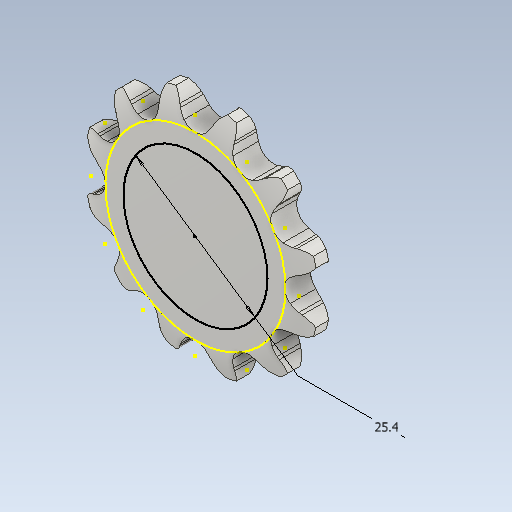
# Autodesk Inventor part: Roller Chain Sprocket2
Saved by Autodesk Inventor 2020 (Build 240168000, 168)
## iProperties
CustomPartVersion: 1
Created: 2021-01-13
Part Number: Roller Chain Sprocket2
Material: Steel
Document SubType Name: Modeling
Designer: lucky
Density: 7.85 g/cm^3
Appearance: Steel
Mass: 35.6372 g
Surface Area: 27.1032 cm^2
Volume: 4.53977 cm^3
Author: lucky
Autodesk Inventor part; units mm, degrees
ref_plane "YZ Plane" through (0, 0, 0) normal (1, 0, 0) x (0, 1, 0)
ref_plane "XZ Plane" through (0, 0, 0) normal (0, 1, 0) x (-1, 0, 0)
sketch "Theoretical Tooth Profile" plane through (0, 0, 0) normal (0, 0, 1) x (1, 0, 0)
  circle A0 centre (0, 0) radius 18.4009 construction
  line L0 (0, 0) -> (0, 18.4009) construction
  line L1 (0, 0) -> (9.2004, 15.9356) construction
  circle A1 centre (0, 0) radius 20.6314
  arc A2 (-1.9847, 16.7356) -> (1.9847, 16.7356) centre (0, 18.4009) ccw
  line L2 (0, 18.4009) -> (9.2004, 15.9356) construction
  line L3 (0, 18.4009) -> (3.1132, 21.0132) construction
  line L4 (3.1132, 21.0132) -> (-2.8337, 18.0265) construction
  arc A3 (4.5324, 20.1274) -> (3.0586, 18.4742) centre (6.8697, 16.5602) ccw
  arc A4 (-3.0586, 18.4742) -> (-4.5324, 20.1274) centre (-6.8697, 16.5602) ccw
  line L5 (-6.8697, 16.5602) -> (-3.0586, 18.4742) construction
  arc A5 (-2.8337, 18.0265) -> (-1.9847, 16.7356) centre (3.1132, 21.0132) ccw
  line L6 (-2.8337, 18.0265) -> (-3.0586, 18.4742)
  arc A6 (1.9847, 16.7356) -> (2.8337, 18.0265) centre (-3.1132, 21.0132) ccw
  line L7 (3.0586, 18.4742) -> (2.8337, 18.0265)
  line L8 (0, 0) -> (5.3398, 19.9284) construction
  point P0 (4.6002, 17.1683)
  dimension "d0" = 36.8018
  dimension "d2" = 30
  dimension "d3" = 2.5908
  dimension "d10" = 130
  dimension "d11" = 13.333
  dimension "d12" = 4.064
  dimension "d13" = 6.6548
  dimension "d14" = 7.112
  dimension "d23" = 2.8575
  constraints: 18 end point, 15 point on circle, 7 centre point, 3 coincident, 3 point on line, 3 symmetric about line, 3 tangent, 1 equal radius, 1 midpoint, 1 parallel, 1 vertical, 1 other
  measures "d0" diameter of A0
  measures "d2" angle of L1 L0
  measures "d3" radius of A2
  measures "d10" angle of L3 L0
  measures "d11" angle of L4 L3
  measures "d12" distance of L2.start L3.end
  measures "d13" distance of L3.end L4.end
  measures "d14" distance of A3.centre L0.end
  measures "d23" distance from line of L8.end L2
sketch "Tooth Profile" plane through (0, 0, 0) normal (0, 0, 1) x (1, 0, 0)
  arc A0 (-2.3714, 17.3575) -> (2.3714, 17.3575) centre (0, 18.4009) ccw
  arc A1 (4.3652, 20.1643) -> (2.3714, 17.3575) centre (10.183, 13.9202) ccw
  arc A2 (-2.3714, 17.3575) -> (-4.3652, 20.1643) centre (-10.183, 13.9202) ccw
  line L0 (0, 0) -> (0, 18.4009) construction
  line L1 (0, 18.4009) -> (2.3714, 17.3575) construction
  line L2 (0, 18.4009) -> (-2.3714, 17.3575) construction
  circle A3 centre (0, 0) radius 20.6314 projected
  dimension "d44" = 132.5
  dimension "d45" = 8.5344
  dimension "d46" = 2.5908
  constraints: 9 point on circle, 6 end point, 3 centre point, 2 tangent, 1 coincident, 1 equal radius, 1 vertical, 1 other
  measures "d44" angle of L2 L1
  measures "d45" radius of A1
  measures "d46" radius of A0
sketch "Section Profile" plane through (0, 0, 0) normal (1, 0, 0) x (0, 1, 0)
  line L0 (20.6314, 0) -> (-20.6314, 0) projected
  line L1 (12.2494, 2.2967) -> (-12.2494, 2.2967)
  line L2 (-12.2494, 2.2967) -> (-12.2494, -2.2967)
  line L3 (-12.2494, -2.2967) -> (12.2494, -2.2967)
  line L4 (12.2494, -2.2967) -> (12.2494, 2.2967)
  line L5 (12.2494, 2.2967) -> (20.6314, 2.2967) construction
  line L6 (20.6314, 2.2967) -> (20.6314, -2.2967) construction
  line L7 (20.6314, -2.2967) -> (12.2494, -2.2967) construction
  line L8 (12.2494, -2.2967) -> (12.2494, 2.2967)
  arc A0 (20.6314, 1.106) -> (15.8677, 2.2967) centre (15.8677, -7.8284) ccw
  arc A1 (15.8677, -2.2967) -> (20.6314, -1.106) centre (15.8677, 7.8284) ccw
  line L9 (15.8677, 2.2967) -> (0, 2.2967)
  line L10 (0, 2.2967) -> (0, -2.2967)
  line L11 (0, -2.2967) -> (15.8677, -2.2967)
  line L12 (0, 2.2967) -> (0, -2.2967)
  line L13 (20.6314, 1.106) -> (20.6314, -1.106)
  point P0 (0, 0)
  point P1 (0, 0)
  dimension "d30" = 4.5933
  dimension "d31" = 24.4988
  dimension "d32" = 4.5933
  dimension "d33" = 1.1906
  dimension "d34" = 10.1251
  dimension "d43" = 2.2967
  constraints: 26 end point, 7 midpoint, 5 perpendicular, 4 parallel, 4 point on circle, 3 point on line, 3 symmetric about line, 2 centre point, 2 horizontal, 2 tangent, 1 collinear, 1 other
  measures "d30" distance between parallel lines of L7 L5
  measures "d31" distance between parallel lines of L2 L4
  measures "d32" distance between parallel lines of L3 L1
  measures "d33" distance from line of L13.start L5
  measures "d34" radius of A0
  measures "d43" distance between parallel lines of L3 L0
revolve "Shroud" add sketch "Section Profile" angle 360 about axis through (0, 0, 2.2967) along (0, 0, -1) contours L10 L3 L2 L0 | L0 L2 L1 L10
revolve "Strand" add sketch "Section Profile" angle 360 about axis through (0, 0, 2.2967) along (0, 0, -1) contours L13 A1 L11 L4 L0 | L0 L4 L9 A0 L13 | L4 L3 L10 L0 | L0 L10 L1 L4
pattern_of_one "Strand Pattern"
extrude "Theoretical Tooth" cut sketch "Theoretical Tooth Profile" along normal through all both and the other way through all contours A3 L7 A6 A2 A5 L6 A4 A1 picked at (-0.5073, 18.0155)
extrude "Tooth" [suppressed]
pattern_circular "Tooth Pattern" count 12 over 360 about axis through (0, 0, -10) along (0, 0, 1) of "Theoretical Tooth"
ref_plane "Timing Plane" through (0, 18.4009, 0) normal (1, 0, 0) x (0, 1, 0)
sketch "Sketch4" plane through (0, 18.4009, 2.2967) normal (0, 0, 1) x (1, 0, 0)
  arc A0 (7.4929, -4.4138) -> (8.3667, -4.9182) centre (9.2004, -2.4653) ccw projected
  arc A1 (7.4929, -4.4138) -> (0.5045, -2.5412) centre (0, -18.4009) ccw projected
  arc A2 (-0.5045, -2.5412) -> (0.5045, -2.5412) centre (0, 0) ccw projected
  arc A3 (-0.5045, -2.5412) -> (-7.4929, -4.4138) centre (0, -18.4009) ccw projected
  arc A4 (-8.3667, -4.9182) -> (-7.4929, -4.4138) centre (-9.2004, -2.4653) ccw projected
  arc A5 (-8.3667, -4.9182) -> (-13.4826, -10.0341) centre (0, -18.4009) ccw projected
  arc A6 (-13.9871, -10.9079) -> (-13.4826, -10.0341) centre (-15.9356, -9.2004) ccw projected
  arc A7 (-13.9871, -10.9079) -> (-15.8597, -17.8964) centre (0, -18.4009) ccw projected
  arc A8 (-15.8597, -18.9054) -> (-15.8597, -17.8964) centre (-18.4009, -18.4009) ccw projected
  arc A9 (-15.8597, -18.9054) -> (-13.9871, -25.8938) centre (0, -18.4009) ccw projected
  arc A10 (-13.4826, -26.7676) -> (-13.9871, -25.8938) centre (-15.9356, -27.6013) ccw projected
  arc A11 (-13.4826, -26.7676) -> (-8.3667, -31.8835) centre (0, -18.4009) ccw projected
  arc A12 (-7.4929, -32.388) -> (-8.3667, -31.8835) centre (-9.2004, -34.3365) ccw projected
  arc A13 (-7.4929, -32.388) -> (-0.5045, -34.2606) centre (0, -18.4009) ccw projected
  arc A14 (0.5045, -34.2606) -> (-0.5045, -34.2606) centre (0, -36.8018) ccw projected
  arc A15 (0.5045, -34.2606) -> (7.4929, -32.388) centre (0, -18.4009) ccw projected
  arc A16 (8.3667, -31.8835) -> (7.4929, -32.388) centre (9.2004, -34.3365) ccw projected
  arc A17 (8.3667, -31.8835) -> (13.4826, -26.7676) centre (0, -18.4009) ccw projected
  arc A18 (13.9871, -25.8938) -> (13.4826, -26.7676) centre (15.9356, -27.6013) ccw projected
  arc A19 (13.9871, -25.8938) -> (15.8597, -18.9054) centre (0, -18.4009) ccw projected
  arc A20 (15.8597, -17.8964) -> (15.8597, -18.9054) centre (18.4009, -18.4009) ccw projected
  arc A21 (15.8597, -17.8964) -> (13.9871, -10.9079) centre (0, -18.4009) ccw projected
  arc A22 (13.4826, -10.0341) -> (13.9871, -10.9079) centre (15.9356, -9.2004) ccw projected
  arc A23 (13.4826, -10.0341) -> (8.3667, -4.9182) centre (0, -18.4009) ccw projected
  circle A24 centre (0, -18.4009) radius 12.7
  dimension "d51" = 25.4
  constraints: 1 centre point, 1 coincident
  measures "d51" diameter of A24
equation "\"d3\" = 0.5 * da_Dr + da_SC"
equation "\"d12\" = 0.8 * da_Dr"
equation "\"d13\" = 1.3 * da_Dr + da_SC"
equation "\"d14\" = 1.4 * da_Dr"
equation "\"d23\" = da_Ha"
equation "\"d44\" = da_Alfa"
equation "\"d45\" = da_Re"
equation "\"d46\" = da_Ri"
equation "\"d30\" = da_Bf"
equation "\"d31\" = da_Ds"
equation "\"d32\" = da_Bs"
equation "\"d33\" = da_Ba"
equation "\"d34\" = da_Rx"
equation "\"d40\" = da_pt"
equation "\"form_type\" = 0"
equation "\"da_p\" = 9.525"
equation "\"da_Dr\" = 5.08"
equation "\"da_SC\" = 0.0508"
equation "\"da_Ha\" = 2.8575"
equation "\"da_pt\" = 10.1346"
equation "\"da_Bf\" = 4.59334"
equation "\"da_Ba\" = 1.19063"
equation "\"da_Rx\" = 10.12508"
equation "\"da_Ra\" = 0.381"
equation "\"da_Bs\" = 4.59334"
equation "\"da_Ds\" = 24.49878"
equation "\"da_Re\" = 8.5344"
equation "\"da_Ri\" = 2.5908"
equation "\"da_Alfa\" = 132.5deg"
body "Solid1"
